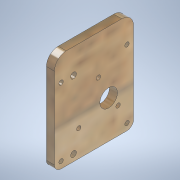
# Autodesk Inventor part: ハンド_モータパネル
Saved by Autodesk Inventor 2020.3 (Build 243373000, 373)
## iProperties
Created: 2020-05-31
Part Number: ハンド_モータパネル
Material: 木材 (カエデ材)
Document SubType Name: Modeling
Designer: totot
Mass: 13.2488 g
Surface Area: 120.842 cm^2
Volume: 19.7744 cm^3
Density: 0.67 g/cm^3
Appearance: ナチュラル カエデ材 - 光沢 濃い着色
Author: totot
Autodesk Inventor part; units mm, degrees
ref_plane "YZ Plane" through (0, 0, 0) normal (1, 0, 0) x (0, 1, 0)
ref_plane "XZ Plane" through (0, 0, 0) normal (0, 1, 0) x (-1, 0, 0)
ref_plane "XY Plane" through (0, 0, 0) normal (0, 0, 1) x (1, 0, 0)
sketch "スケッチ1" plane through (0, 0, 0) normal (1, 0, 0) x (0, 1, 0)
  line L0 (0, 0) -> (-55.5, 0)
  line L1 (-55.5, 0) -> (-55.5, -54)
  line L2 (-55.5, -54) -> (0, -54)
  line L3 (0, -54) -> (0, 0)
  dimension "d0" = 55.5
  dimension "d1" = 54
  constraints: 8 end point, 2 parallel, 1 horizontal, 1 perpendicular
  measures "d0" distance of L2.end L1.end
  measures "d1" distance of L1.end L0.end
extrude "押し出し1" add sketch "スケッチ1" along normal blind 5.5
sketch "スケッチ2" plane through (5.5, 0, 0) normal (1, 0, 0) x (0, 0, -1)
  line L0 (54, 0) -> (0, 0) projected
  line L1 (54, -55.5) -> (54, 0) projected
  line L2 (0, -55.5) -> (54, -55.5) projected
  line L3 (0, 0) -> (0, -55.5) projected
  point P0 (4.5, -4.5)
  point P1 (49.5, -4.5)
  point P2 (4.5, -51)
  point P3 (49.5, -51)
  dimension "d4" = 4.5
  dimension "d5" = 4.5
  dimension "d6" = 4.5
  dimension "d7" = 4.5
  dimension "d8" = 4.5
  dimension "d9" = 4.5
  dimension "d10" = 4.5
  dimension "d11" = 4.5
  measures "d4" distance from line of point (4.5, -4.5) L0
  measures "d5" distance from line of point (49.5, -4.5) L1
  measures "d6" distance from line of point (49.5, -4.5) L0
  measures "d7" distance from line of point (49.5, -51) L2
  measures "d8" distance from line of point (49.5, -51) L1
  measures "d9" distance from line of L2 point (4.5, -51)
  measures "d10" distance from line of L3 point (4.5, -51)
  measures "d11" distance from line of L3 point (4.5, -4.5)
hole "穴1" at (5.5, -4.5, -4.5) at (5.5, -4.5, -49.5) at (5.5, -51, -4.5) at (5.5, -51, -49.5) direction (-1, 0, 0) diameter 3 end through all
sketch "スケッチ3" plane through (5.5, 0, 0) normal (1, 0, 0) x (0, 0, -1)
  line L0 (54, 0) -> (0, 0) projected
  line L1 (0, -55.5) -> (54, -55.5) projected
  circle A0 centre (4.5, -51) radius 1.5 projected
  circle A1 centre (4.5, -4.5) radius 1.5 projected
  point P0 (13, -4.5)
  point P1 (13, -51)
  dimension "d19" = 4.5
  dimension "d20" = 4.5
  dimension "d21" = 8.5
  dimension "d22" = 8.5
  measures "d19" distance from line of point (13, -4.5) L0
  measures "d20" distance from line of point (13, -51) L1
  measures "d21" distance of A0.centre point (13, -51)
  measures "d22" distance of point (13, -4.5) A1.centre
hole "穴2" at (5.5, -4.5, -13) at (5.5, -51, -13) direction (-1, 0, 0) diameter 4 end through all
sketch "スケッチ4" plane through (0, 0, 0) normal (-1, 0, 0) x (0, 0, 1)
  line L0 (-30, -14.25) -> (-30, -29.75)
  line L1 (-30, -14.25) -> (-14.5, -14.25) construction
  line L2 (-30, -29.75) -> (-16.5766, -37.5)
  line L3 (-30, -29.75) -> (-43.4234, -37.5)
  line L4 (-30, -29.75) -> (-14.5, -29.75) construction
  circle A0 centre (-43.4234, -37.5) radius 1.5
  circle A1 centre (-16.5766, -37.5) radius 1.5
  circle A2 centre (-30, -14.25) radius 1.5
  circle A3 centre (-37, -29.75) radius 6
  line L5 (0, -55.5) -> (-54, -55.5) projected
  line L6 (-54, 0) -> (0, 0) projected
  line L7 (-54, -55.5) -> (-54, 0) projected
  dimension "d30" = 15.5
  dimension "d31" = 90
  dimension "d32" = 15.5
  dimension "d33" = 120
  dimension "d34" = 15.5
  dimension "d35" = 150
  dimension "d36" = 3
  dimension "d37" = 3
  dimension "d38" = 3
  dimension "d42" = 12
  dimension "d43" = 7
  dimension "d44" = 0
  dimension "d47" = 25.75
  dimension "d48" = 55.5
  dimension "d49" = 24
  constraints: 10 end point, 4 centre point, 3 coincident, 2 equal length, 2 horizontal, 1 vertical
  measures "d30" distance of L0.start L0.end
  measures "d31" angle of L0 L1
  measures "d32" distance of L0.end L2.end
  measures "d33" angle of L2 L0
  measures "d34" distance of L0.end L3.end
  measures "d35" angle of L3 L4
  measures "d36" diameter of A0
  measures "d37" diameter of A1
  measures "d38" diameter of A2
  measures "d42" diameter of A3
  measures "d43" distance of L0.end A3.centre
  measures "d44" vertical distance of L0.end A3.centre
  measures "d47" distance from line of L0.end L5
  measures "d48" distance between parallel lines of L6 L5
  measures "d49" distance from line of L0.end L7
extrude "押し出し3" cut sketch "スケッチ4" against normal blind 10
sketch "スケッチ5" plane through (0, 0, 0) normal (0, 1, 0) x (1, 0, 0)
  line L0 (0, 0) -> (5.5, 0) projected
  line L1 (5.5, 0) -> (5.5, 54) projected
  line L2 (0, 0) -> (5.5, 0)
  line L3 (5.5, 0) -> (5.5, 54)
  line L4 (5.5, 54) -> (0, 54)
  line L5 (0, 54) -> (0, 0)
  constraints: 8 end point, 2 parallel, 1 horizontal, 1 perpendicular
extrude "押し出し4" add sketch "スケッチ5" along normal blind 25
fillet "フィレット2" radius 8 2 edges at (2.75, 25, -54) (2.75, 25, 0)
fillet "フィレット3" radius 4.5 2 edges at (2.75, -55.5, -54) (2.75, -55.5, 0)
sketch "スケッチ6" plane through (0, 0, 0) normal (-1, 0, 0) x (0, 0, 1)
  line L0 (-46, 25) -> (-8, 25) projected
  circle A0 centre (-37, -29.75) radius 6 projected
  line L1 (-54, -51) -> (-54, 17) projected
  point P0 (0, 0)
  point P1 (-37, 18)
  dimension "d55" = 7
  dimension "d56" = 17
  dimension "d57" = 17
  measures "d55" distance from line of point (-37, 18) L0
  measures "d56" distance from line of A0.centre L1
  measures "d57" distance from line of point (-37, 18) L1
hole "穴3" at (0, 18, -37) direction (1, 0, 0) diameter 8 end through all
sketch "スケッチ7" plane through (0, 0, 0) normal (-1, 0, 0) x (0, 0, 1)
  line L0 (-46, 25) -> (-8, 25) projected
  line L1 (0, -51) -> (0, 17) projected
  point P0 (0, 0)
  point P1 (-10, 15)
  point P2 (-15, 15)
  point P3 (-20, 15)
  point P4 (-25, 15)
  point P5 (-10, 10)
  point P6 (-15, 10)
  point P7 (-20, 10)
  point P8 (-25, 10)
  point P9 (-10, 5)
  point P10 (-15, 5)
  point P11 (-20, 5)
  point P12 (-25, 5)
  point P13 (-10, 0)
  point P14 (-15, 0)
  point P15 (-20, 0)
  point P16 (-25, 0)
  point P17 (-10, 20)
  point P18 (-15, 15)
  point P19 (-15, 20)
  point P20 (-20, 15)
  point P21 (-20, 20)
  point P22 (-25, 15)
  point P23 (-25, 20)
  point P24 (-30, 15)
  point P25 (-30, 20)
  point P26 (-5, 15)
  point P27 (-10, 10)
  point P28 (-5, 10)
  point P29 (-10, 5)
  point P30 (-5, 5)
  point P31 (-10, 0)
  point P32 (-5, 0)
  point P33 (-30, 10)
  point P34 (-35, 10)
  point P35 (-40, 10)
  point P36 (-45, 10)
  point P37 (-25, 5)
  point P38 (-30, 5)
  point P39 (-35, 5)
  point P40 (-40, 5)
  point P41 (-45, 5)
  point P42 (-25, 0)
  point P43 (-30, 0)
  point P44 (-35, 0)
  point P45 (-40, 0)
  point P46 (-45, 0)
  dimension "d65" = 10
  dimension "d66" = 10
  dimension "d69" = 5
  dimension "d72" = 5
  dimension "d77" = 5
  dimension "d80" = 5
  dimension "d85" = 5
  dimension "d88" = 5
  dimension "d93" = 5
  dimension "d96" = 5
  constraints: 4 horizontal, 4 vertical, 45 other
  measures "d65" distance from line of L0 point (-10, 15)
  measures "d66" distance from line of L1 point (-10, 15)
  measures "d69" distance of point (-10, 15) point (-15, 15)
  measures "d72" distance of point (-10, 15) point (-10, 10)
  measures "d77" distance of point (-10, 15) point (-10, 20)
  measures "d80" distance of point (-10, 15) point (-15, 15)
  measures "d85" distance of point (-10, 15) point (-5, 15)
  measures "d88" distance of point (-10, 15) point (-10, 10)
  measures "d93" distance of point (-25, 10) point (-30, 10)
  measures "d96" distance of point (-25, 10) point (-25, 5)
hole "穴4" at (0, 15, -10) at (0, 15, -15) at (0, 15, -20) at (0, 15, -25) at (0, 10, -10) at (0, 10, -15) at (0, 10, -20) at (0, 10, -25) at (0, 5, -10) at (0, 5, -15) at (0, 5, -20) at (0, 5, -25) at (0, 0, -10) at (0, 0, -15) at (0, 0, -20) at (0, 0, -25) at (0, 20, -10) at (0, 20, -15) at (0, 20, -20) at (0, 20, -25) at (0, 15, -30) at (0, 20, -30) at (0, 15, -5) at (0, 10, -5) at (0, 5, -5) at (0, 0, -5) at (0, 10, -30) at (0, 10, -35) at (0, 10, -40) at (0, 10, -45) at (0, 5, -30) at (0, 5, -35) at (0, 5, -40) at (0, 5, -45) at (0, 0, -30) at (0, 0, -35) at (0, 0, -40) at (0, 0, -45) direction (1, 0, 0) diameter 4 end through all
equation "\"d5\" = d4"
equation "\"d6\" = d5"
equation "\"d7\" = d6"
equation "\"d8\" = d6"
equation "\"d9\" = d7"
equation "\"d10\" = d8"
equation "\"d11\" = d4"
equation "\"d20\" = d19"
equation "\"d22\" = d21"
equation "\"d57\" = d56"
equation "\"d66\" = d65"
